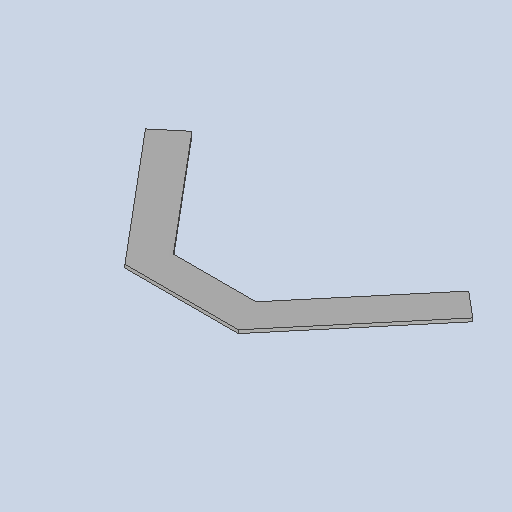
# Autodesk Inventor part: ДМФ 044 фланец лотка
Saved by Autodesk Inventor 2024.2 (Build 282272000, 272)
## iProperties
Created: 2024-05-14
Part Number: ДМФ 044 фланец лотка
Material: Generic
Document SubType Name: Sheet Metal
Designer: admin
Density: 1 g/cm^3
Sheet Metal Rule: Default_mm
Appearance: Default
Author: admin
Autodesk Inventor part; units mm, degrees
ref_plane "YZ Plane" through (0, 0, 0) normal (1, 0, 0) x (0, 1, 0)
ref_plane "XZ Plane" through (0, 0, 0) normal (0, 1, 0) x (-1, 0, 0)
ref_plane "XY Plane" through (0, 0, 0) normal (0, 0, 1) x (1, 0, 0)
sketch "Sketch1" plane through (0, 0, 0) normal (0, 0, 1) x (1, 0, 0)
  line L0 (-25, 0) -> (25, 0)
  line L1 (25, 0) -> (83.737, 70)
  line L2 (83.737, 70) -> (99.0579, 57.1442)
  line L3 (99.0579, 57.1442) -> (34.3262, -20)
  line L4 (34.3262, -20) -> (-34.3262, -20)
  line L5 (-34.3262, -20) -> (-99.0579, 57.1442)
  line L6 (-99.0579, 57.1442) -> (-83.737, 70)
  line L7 (-83.737, 70) -> (-25, 0)
  line L8 (0, 0) -> (0, -20) construction
  dimension "d0" = 50
  dimension "d1" = 70
  dimension "d2" = 130
  dimension "d3" = 20
  measures "d0" distance of L0.start L0.end
  measures "d1" distance from line of L0 L6.end
  measures "d2" angle of L0 L7
  measures "d3" distance of L5.end L6.end
extrude "Plate1" add sketch "Sketch1" along normal blind 2
equation "\"d0\" = Лоток_ширина_низ"
equation "\"d1\" = Лоток_высота - Лоток_глубина_выреза"
equation "\"d2\" = Лоток_угол"
equation "\"d4\" = Thickness"
equation "\"BendRadius\" = Thickness"
equation "\"BendReliefWidth\" = Thickness"
equation "\"BendReliefDepth\" = 0.5 * Thickness"
equation "\"CornerReliefSize\" = 4 * Thickness"
equation "\"MinimumRemnant\" = 2 * Thickness"
equation "\"TransitionRadius\" = BendRadius"
equation "\"JacobiRadiusSize\" = BendRadius"
equation "\"GapSize\" = Thickness"
equation "\"Лоток_ширина_низ\" = 50"
equation "\"Лоток_высота\" = 100"
equation "\"Лоток_глубина_выреза\" = 30"
equation "\"Лоток_угол\" = 130deg"
equation "\"Thickness\" = 2"
body "Solid1"
